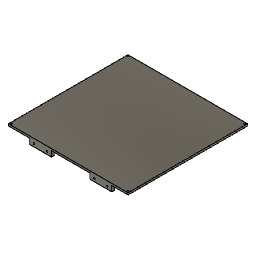
Back of Frame v7 (Autodesk Fusion 360 design; units mm, degrees)
Autodesk Fusion 360 part; units mm, degrees
sketch "Sketch1" plane through (0, 0, 0) normal (0, 0, 1) x (1, 0, 0)
  line L0 (-80, 75) -> (140, 75)
  line L1 (140, 75) -> (140, -145)
  line L2 (140, -145) -> (-80, -145)
  line L3 (-80, -145) -> (-80, 75)
  circle A0 centre (-77.5, 72.5) radius 1.5
  circle A1 centre (137.5, 72.5) radius 1.5
  circle A2 centre (137.5, -142.5) radius 1.5
  circle A3 centre (-77.5, -142.5) radius 1.5
  dimension "d1" = 220
  dimension "d2" = 220
  dimension "d3" = 3
  dimension "d4" = 3
  dimension "d5" = 3
  dimension "d6" = 3
  dimension "d7" = 2.5
  dimension "d8" = 2.5
  dimension "d9" = 2.5
  dimension "d10" = 2.5
  dimension "d11" = 2.5
  dimension "d12" = 2.5
  dimension "d13" = 2.5
  dimension "d14" = 2.5
  constraint horizontal L0
  constraint vertical L1
  constraint horizontal L2
  constraint vertical L3
  measures "d1" distance of L0.start L0.end
  measures "d2" distance of L0.start L2.end
  measures "d3" diameter of A0
  measures "d4" diameter of A1
  measures "d5" diameter of A2
  measures "d6" diameter of A3
  measures "d7" distance of L2 A3.centre
  measures "d8" distance of L3 A3.centre
  measures "d9" distance of L0 A0.centre
  measures "d10" distance of L3 A0.centre
  measures "d11" distance of L0 A1.centre
  measures "d12" distance of L1 A1.centre
  measures "d13" distance of L1 A2.centre
  measures "d14" distance of L2 A2.centre
extrude "Extrude1" add sketch "Sketch1" along normal blind 3.5
sketch "Sketch2" plane through (0, 0, 0) normal (0, 0, -1) x (1, 0, 0)
  circle A0 centre (137.5, 142.5) radius 1.5
  circle A1 centre (137.5, -72.5) radius 1.5
  circle A2 centre (-77.5, -72.5) radius 1.5
  circle A3 centre (-77.5, 142.5) radius 1.5
  line L0 (140, 145) -> (-80, 145)
  line L1 (-80, 145) -> (-80, -75)
  line L2 (-80, -75) -> (140, -75)
  line L3 (140, -75) -> (140, 145)
  line L4 (-41, 145) -> (-1, 145)
  line L5 (-1, 145) -> (-1, 140)
  line L6 (-1, 140) -> (-41, 140)
  line L7 (-41, 140) -> (-41, 145)
  line L8 (70, 145) -> (110, 145)
  line L9 (110, 145) -> (110, 140)
  line L10 (110, 140) -> (70, 140)
  line L11 (70, 140) -> (70, 145)
  dimension "d17" = 5
  dimension "d18" = 5
  dimension "d19" = 40
  dimension "d20" = 40
  dimension "d21" = 30
  dimension "d22" = 39
  constraint horizontal L4
  constraint vertical L5
  constraint horizontal L6
  constraint vertical L7
  constraint coincident L0 L4.start
  constraint horizontal L8
  constraint vertical L9
  constraint horizontal L10
  constraint vertical L11
  constraint coincident L0 L8.start
  measures "d17" distance of L8 L10
  measures "d18" distance of L4 L6
  measures "d19" distance of L5 L7
  measures "d20" distance of L9 L11
  measures "d21" distance of L3 L9
  measures "d22" distance of L1 L7
extrude "Extrude2" add sketch "Sketch2" along normal blind 10 contours L0 L8 L9 L10 L11 | L0 L4 L5 L6 L7
sketch "Sketch3" plane through (0, -145, 0) normal (0, -1, 0) x (1, 0, 0)
  line L0 (110, 0) -> (140, 0)
  line L1 (140, 0) -> (140, 3.5)
  line L2 (140, 3.5) -> (-80, 3.5)
  line L3 (-80, 3.5) -> (-80, 0)
  line L4 (-80, 0) -> (-41, 0)
  line L5 (-41, 0) -> (-41, -10)
  line L6 (-41, -10) -> (-1, -10)
  line L7 (-1, -10) -> (-1, 0)
  line L8 (-1, 0) -> (70, 0)
  line L9 (70, 0) -> (70, -10)
  line L10 (70, -10) -> (110, -10)
  line L11 (110, -10) -> (110, 0)
  circle A0 centre (-33, -5) radius 1.5
  circle A1 centre (-9, -5) radius 1.5
  circle A2 centre (78, -5) radius 1.5
  circle A3 centre (102, -5) radius 1.5
  dimension "d25" = 3
  dimension "d26" = 3
  dimension "d27" = 3
  dimension "d28" = 3
  dimension "d29" = 5
  dimension "d30" = 5
  dimension "d31" = 8
  dimension "d32" = 8
  dimension "d33" = 5
  dimension "d34" = 8
  dimension "d35" = 8
  dimension "d36" = 5
  measures "d25" diameter of A0
  measures "d26" diameter of A1
  measures "d27" diameter of A2
  measures "d28" diameter of A3
  measures "d29" distance of L10 A3.centre
  measures "d30" distance of L10 A2.centre
  measures "d31" distance of L11 A3.centre
  measures "d32" distance of L9 A2.centre
  measures "d33" distance of L6 A1.centre
  measures "d34" distance of L7 A1.centre
  measures "d35" distance of L5 A0.centre
  measures "d36" distance of L6 A0.centre
extrude "Extrude3" cut sketch "Sketch3" against normal blind 5 contours A0 | A1 | A2 | A3
